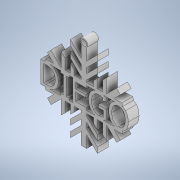
# Autodesk Inventor part: Diego
Saved by Autodesk Inventor 2021 (Build 250183000, 183)
## iProperties
Created: 2020-12-16
Part Number: Diego
Material: Genérico
Document SubType Name: Modeling
Designer: yosaf
Density: 1 g/cm^3
Appearance: Valor por defecto
Author: yosaf
Autodesk Inventor part; units mm, degrees
ref_plane "YZ Plane" through (0, 0, 0) normal (1, 0, 0) x (0, 1, 0)
ref_plane "XZ Plane" through (0, 0, 0) normal (0, 1, 0) x (-1, 0, 0)
ref_plane "XY Plane" through (0, 0, 0) normal (0, 0, 1) x (1, 0, 0)
sketch "Boceto1" plane through (0, 0, 0) normal (0, 1, 0) x (-1, 0, 0)
  point P0 (0, 0)
sketch "Boceto2" plane through (0, 0, 0) normal (0, 0, 1) x (1, 0, 0)
  line L0 (37.5, 0) -> (37.5, 10) construction
  line L1 (36.1421, 10) -> (0, 10)
  line L2 (37.5, 0) -> (37.5, -10) construction
  line L3 (36.1421, 10) -> (36.1421, 12.5) construction
  line L4 (-2.5, 37.5) -> (0, 37.5) construction
  line L5 (2.5, 37.5) -> (2.5, 12.5)
  line L6 (-2.5, 37.5) -> (-2.5, 37.4166)
  line L7 (-2.5, 37.5) -> (-2.5, 29.5) construction
  line L8 (-2.5, 29.5) -> (-9.3227, 36.3227) construction
  line L9 (-2.5, 29.5) -> (7.1487, 29.5) construction
  line L10 (-2.5, 29.5) -> (-2.5, 24.5) construction
  line L11 (2.3244, 29.5) -> (9.1827, 36.3583)
  line L12 (2.3244, 29.5) -> (12.0235, 29.5) construction
  line L13 (2.5, 24.5) -> (12.505, 34.505)
  line L14 (2.5, 12.5) -> (2.5, 14.5) construction
  line L15 (2.5, 14.5) -> (12.505, 24.505)
  line L16 (2.5, 14.5) -> (19.9142, 14.5) construction
  line L17 (12.505, 34.505) -> (12.505, 24.505) construction
  line L18 (2.5, 14.5) -> (2.5, 19.5) construction
  line L19 (2.5, 19.5) -> (9.655, 26.655)
  line L20 (9.1827, 36.3583) -> (12.505, 39.6807)
  line L21 (12.505, 39.6807) -> (12.505, 34.505)
  line L22 (9.655, 26.655) -> (12.505, 29.505)
  line L23 (12.505, 24.505) -> (12.505, 29.505)
  line L24 (12.505, 12.5) -> (12.505, 20.7373)
  line L25 (12.505, 12.5) -> (8.969, 12.5) construction
  line L26 (8.9413, 12.2486) -> (8.9413, 17.1736)
  line L27 (2.5, 37.4166) -> (2.5, 40.7545)
  line L28 (2.5, 40.7545) -> (0, 40.7545)
  line L29 (-2.5, 37.5) -> (-2.5, 37.4166)
  line L30 (12.505, 12.5) -> (17.505, 12.5) construction
  line L31 (12.505, 29.505) -> (26.5274, 43.5274) construction
  line L32 (17.505, 12.5) -> (21.041, 12.5) construction
  line L33 (21.041, 12.5) -> (21.041, 24.5)
  line L34 (21.041, 12.5) -> (27.7806, 19.2396) construction
  line L35 (21.041, 12.5) -> (21.041, 21.5913) construction
  line L36 (21.041, 12.5) -> (30.3882, 21.8472)
  line L37 (30.3882, 21.8472) -> (33.9237, 18.3116)
  arc A0 (36.1421, 10) -> (35.3553, 12.5) centre (0, 0) ccw
  line L38 (2.5, 14.5) -> (18.1273, 30.1273) construction
  line L39 (17.505, 12.5) -> (17.505, 22.0456)
  line L40 (17.505, 20.7373) -> (12.505, 20.7373) construction
  line L41 (12.505, 20.7373) -> (8.9413, 17.1736)
  line L42 (0, 40.7545) -> (0, 10) construction
  line L43 (35.3553, 12.5) -> (0, 12.5)
  line L44 (-2.5, 24.5) -> (-2.5878, 24.5878)
  line L45 (0, 10) -> (-36.142, 10)
  line L46 (0, 40.7545) -> (-2.5, 40.7545)
  line L47 (-2.5, 40.7545) -> (-2.5, 12.5)
  line L48 (-2.5, 12.5) -> (0, 12.5)
  arc A1 (10.5574, 39.7112) -> (12.505, 39.6807) centre (11.546, 40.6397) ccw construction
  line L49 (-2.505, 29.505) -> (-12.7112, 39.7112)
  line L50 (-2.505, 29.505) -> (11.9286, 29.505) construction
  line L51 (-2.5, 19.4405) -> (-12.5645, 29.505)
  line L52 (-2.5, 19.4405) -> (11.7334, 19.4405) construction
  line L53 (-12.5645, 29.505) -> (-12.5645, 24.4414)
  line L54 (-12.5645, 24.4414) -> (-2.5, 14.3769)
  line L55 (-12.5645, 12.5) -> (-2.5, 12.5)
  line L56 (17.505, 22.0456) -> (21.041, 25.5816)
  line L57 (17.505, 22.0456) -> (22.5057, 22.0456) construction
  line L58 (21.041, 25.5816) -> (21.041, 24.5)
  line L59 (-12.5645, 20.7373) -> (-12.5645, 20.7373)
  line L60 (-12.5645, 20.7373) -> (-7.5226, 20.7373) construction
  line L61 (0, 12.5) -> (-35.355, 12.5)
  arc A2 (-35.3554, 12.4999) -> (-36.1419, 10) centre (0.0007, 0.0021) ccw
  line L62 (-12.5806, 20.7428) -> (-9.0285, 17.1736)
  line L63 (-12.5645, 20.7373) -> (-17.5614, 12.5) construction
  line L64 (-17.5614, 12.5) -> (-17.5645, 22.0456)
  line L65 (-17.5645, 22.0456) -> (-21.1198, 25.6009)
  line L66 (-17.5645, 22.0456) -> (-12.5366, 22.0456) construction
  line L67 (-21.1198, 25.6009) -> (-21.1198, 12.5)
  line L68 (33.9237, 18.3116) -> (-56.2408, 18.3116) construction
  line L69 (30.1897, 22.0456) -> (-56.2408, 22.0456) construction
  line L70 (33.9237, 18.3116) -> (33.178, 17.4812)
  line L71 (33.9237, 18.3116) -> (28.1121, 12.5)
  line L72 (33.9237, 18.3116) -> (42.1426, 18.3116) construction
  line L73 (-21.1198, 12.5) -> (-30.6654, 22.0456)
  line L74 (-21.1198, 12.5) -> (-7.6202, 12.5) construction
  line L75 (-30.6654, 22.0456) -> (-33.9907, 18.3116)
  line L76 (-21.1198, 12.5) -> (-25.4451, 12.5) construction
  line L77 (-28.1908, 12.5) -> (-33.9907, 18.3116)
  line L78 (-25.4451, 12.5) -> (-25.4451, 10)
  line L79 (-2.5, 12.5) -> (-2.5, 10)
  line L80 (-12.5645, 12.5) -> (-12.5645, 10)
  line L81 (2.5, 12.5) -> (2.5, 10)
  line L82 (17.505, 12.5) -> (17.505, 10)
  line L83 (28.1121, 12.5) -> (28.1121, 10)
  line L84 (-28.1908, 12.5) -> (-28.1908, 10)
  line L85 (-36.1419, 10) -> (-35.3553, 12.5)
  line L86 (-35.3553, 12.5) -> (-28.1908, 12.5)
  line L87 (-36.1419, 10) -> (-28.1908, 10)
  line L88 (-12.5806, 20.7428) -> (-8.8604, 20.7373) construction
  line L89 (-12.5645, 24.4414) -> (-12.5645, 20.7373) construction
  line L90 (-12.5645, 20.7373) -> (-12.5645, 12.5)
  line L91 (8.9413, 17.1736) -> (-10.7205, 17.1736) construction
  line L92 (-12.5645, 12.5) -> (-9.0285, 12.5) construction
  line L93 (-9.0285, 12.4865) -> (-9.0285, 17.1736)
  line L94 (-9.0285, 12.4865) -> (-4.3415, 12.4865) construction
  line L95 (-12.5645, 12.5) -> (-17.5645, 12.5) construction
  line L96 (-17.5645, 12.5) -> (-21.1005, 12.5) construction
  line L97 (12.505, 39.6807) -> (-23.2825, 39.6807) construction
  line L98 (12.505, 39.6807) -> (48.2925, 39.6807) construction
  line L99 (-12.6807, 39.6807) -> (-12.6807, 31.9273) construction
  line L100 (-12.6807, 39.6807) -> (-4.9273, 39.6807) construction
  line L101 (2.5, 24.5) -> (-2.5, 24.5) construction
  line L102 (-2.5, 24.5) -> (-12.6807, 34.6807)
  line L103 (-12.6807, 39.6807) -> (-12.6807, 34.6807)
  line L104 (-2.5, 29.5) -> (-2.5, 24.5)
  line L105 (-12.6807, 39.6807) -> (-12.6807, 34.6807)
  line L106 (-12.6807, 34.6807) -> (-2.5, 24.5)
  line L107 (-2.5, 24.5) -> (-2.5, 29.5)
  line L108 (-5.3887, 32.3887) -> (-7.0094, 29.0094)
  line L109 (-9.8604, 36.8604) -> (-11.5, 33.5)
  line L110 (-3.3099, 30.3099) -> (-3.3099, 25.3099)
  line L111 (-3.3099, 27) -> (-2.5, 27)
  line L112 (-3.3099, 28.6951) -> (-2.5, 28.6951)
  line L113 (-2.5, 29.5) -> (-3.3099, 30.3099)
  line L114 (-3.3099, 28.6951) -> (-2.5, 28.6951)
  line L115 (-62.0182, 0.0021) -> (57.1522, 0.0021) construction
  line L116 (36.1421, -9.9958) -> (0, -9.9958)
  line L117 (36.1421, -9.9958) -> (36.1421, -12.4958) construction
  line L118 (-2.5, -37.4958) -> (0, -37.4958) construction
  line L119 (2.5, -37.4958) -> (2.5, -12.4958)
  line L120 (-2.5, -37.4958) -> (-2.5, -37.4124)
  line L121 (-2.5, -37.4958) -> (-2.5, -29.4958) construction
  line L122 (-2.5, -29.4958) -> (-9.3227, -36.3185) construction
  line L123 (-2.5, -29.4958) -> (7.1487, -29.4958) construction
  line L124 (-2.5, -29.4958) -> (-2.5, -24.4958) construction
  line L125 (2.3244, -29.4958) -> (9.1827, -36.3541)
  line L126 (2.3244, -29.4958) -> (12.0235, -29.4958) construction
  line L127 (2.5, -24.4958) -> (12.505, -34.5008)
  line L128 (2.5, -12.4958) -> (2.5, -14.4958) construction
  line L129 (2.5, -14.4958) -> (12.505, -24.5008)
  line L130 (2.5, -14.4958) -> (19.9142, -14.4958) construction
  line L131 (12.505, -34.5008) -> (12.505, -24.5008) construction
  line L132 (2.5, -14.4958) -> (2.5, -19.4958) construction
  line L133 (2.5, -19.4958) -> (9.655, -26.6507)
  line L134 (9.1827, -36.3541) -> (12.505, -39.6765)
  line L135 (12.505, -39.6765) -> (12.505, -34.5008)
  line L136 (9.655, -26.6507) -> (12.505, -29.5008)
  line L137 (12.505, -24.5008) -> (12.505, -29.5008)
  line L138 (12.505, -12.4958) -> (12.505, -20.7331)
  line L139 (12.505, -12.4958) -> (8.969, -12.4958) construction
  line L140 (8.9413, -12.2444) -> (8.9413, -17.1694)
  line L141 (2.5, -37.4124) -> (2.5, -40.7503)
  line L142 (2.5, -40.7503) -> (0, -40.7503)
  line L143 (-2.5, -37.4958) -> (-2.5, -37.4124)
  line L144 (12.505, -12.4958) -> (17.505, -12.4958) construction
  line L145 (12.505, -29.5008) -> (26.5274, -43.5232) construction
  line L146 (17.505, -12.4958) -> (21.041, -12.4958) construction
  line L147 (21.041, -12.4958) -> (21.041, -24.4958)
  line L148 (21.041, -12.4958) -> (27.7806, -19.2354) construction
  line L149 (21.041, -12.4958) -> (21.041, -21.5871) construction
  line L150 (21.041, -12.4958) -> (30.3882, -21.843)
  line L151 (30.3882, -21.843) -> (33.9237, -18.3074)
  arc A3 (35.3553, -12.4958) -> (36.1421, -9.9958) centre (0, 0.0042) ccw
  line L152 (2.5, -14.4958) -> (18.1273, -30.1231) construction
  line L153 (17.505, -12.4958) -> (17.505, -22.0414)
  line L154 (17.505, -20.7331) -> (12.505, -20.7331) construction
  line L155 (12.505, -20.7331) -> (8.9413, -17.1694)
  line L156 (0, -40.7503) -> (0, -9.9958) construction
  line L157 (35.3553, -12.4958) -> (0, -12.4958)
  line L158 (-2.5, -24.4958) -> (-2.5878, -24.5836)
  line L159 (0, -9.9958) -> (-36.142, -9.9958)
  line L160 (0, -40.7503) -> (-2.5, -40.7503)
  line L161 (-2.5, -40.7503) -> (-2.5, -12.4958)
  line L162 (-2.5, -12.4958) -> (0, -12.4958)
  arc A4 (12.505, -39.6765) -> (10.5574, -39.707) centre (11.546, -40.6355) ccw construction
  line L163 (-2.505, -29.5008) -> (-12.7112, -39.707)
  line L164 (-2.505, -29.5008) -> (11.9286, -29.5008) construction
  line L165 (-2.5, -19.4363) -> (-12.5645, -29.5008)
  line L166 (-2.5, -19.4363) -> (11.7334, -19.4363) construction
  line L167 (-12.5645, -29.5008) -> (-12.5645, -24.4372)
  line L168 (-12.5645, -24.4372) -> (-2.5, -14.3727)
  line L169 (-12.5645, -12.4958) -> (-2.5, -12.4958)
  line L170 (17.505, -22.0414) -> (21.041, -25.5774)
  line L171 (17.505, -22.0414) -> (22.5057, -22.0414) construction
  line L172 (21.041, -25.5774) -> (21.041, -24.4958)
  line L173 (-12.5645, -20.7331) -> (-12.5645, -20.7331)
  line L174 (-12.5645, -20.7331) -> (-7.5226, -20.7331) construction
  line L175 (0, -12.4958) -> (-35.355, -12.4958)
  arc A5 (-36.1419, -9.9958) -> (-35.3554, -12.4957) centre (0.0007, 0.0021) ccw
  line L176 (-12.5806, -20.7386) -> (-9.0285, -17.1694)
  line L177 (-12.5645, -20.7331) -> (-17.5614, -12.4958) construction
  line L178 (-17.5614, -12.4958) -> (-17.5645, -22.0414)
  line L179 (-17.5645, -22.0414) -> (-21.1198, -25.5967)
  line L180 (-17.5645, -22.0414) -> (-12.5366, -22.0414) construction
  line L181 (-21.1198, -25.5967) -> (-21.1198, -12.4958)
  line L182 (33.9237, -18.3074) -> (33.178, -17.477)
  line L183 (33.9237, -18.3074) -> (28.1121, -12.4958)
  line L184 (33.9237, -18.3074) -> (42.1426, -18.3074) construction
  line L185 (-21.1198, -12.4958) -> (-30.6654, -22.0414)
  line L186 (-21.1198, -12.4958) -> (-7.6202, -12.4958) construction
  line L187 (-30.6654, -22.0414) -> (-33.9907, -18.3074)
  line L188 (-21.1198, -12.4958) -> (-25.4451, -12.4958) construction
  line L189 (-28.1908, -12.4958) -> (-33.9907, -18.3074)
  line L190 (-25.4451, -12.4958) -> (-25.4451, -9.9958)
  line L191 (-2.5, -12.4958) -> (-2.5, -9.9958)
  line L192 (-12.5645, -12.4958) -> (-12.5645, -9.9958)
  line L193 (2.5, -12.4958) -> (2.5, -9.9958)
  line L194 (17.505, -12.4958) -> (17.505, -9.9958)
  line L195 (28.1121, -12.4958) -> (28.1121, -9.9958)
  line L196 (-28.1908, -12.4958) -> (-28.1908, -9.9958)
  line L197 (-36.1419, -9.9958) -> (-35.3553, -12.4958)
  line L198 (-35.3553, -12.4958) -> (-28.1908, -12.4958)
  line L199 (-36.1419, -9.9958) -> (-28.1908, -9.9958)
  line L200 (-12.5806, -20.7386) -> (-8.8604, -20.7331) construction
  line L201 (-12.5645, -24.4372) -> (-12.5645, -20.7331) construction
  line L202 (-12.5645, -20.7331) -> (-12.5645, -12.4958)
  line L203 (8.9413, -17.1694) -> (-10.7205, -17.1694) construction
  line L204 (-12.5645, -12.4958) -> (-9.0285, -12.4958) construction
  line L205 (-9.0285, -12.4823) -> (-9.0285, -17.1694)
  line L206 (-9.0285, -12.4823) -> (-4.3415, -12.4823) construction
  line L207 (-12.5645, -12.4958) -> (-17.5645, -12.4958) construction
  line L208 (-17.5645, -12.4958) -> (-21.1005, -12.4958) construction
  line L209 (12.505, -39.6765) -> (-23.2825, -39.6765) construction
  line L210 (-12.6807, -39.6765) -> (-12.6807, -31.9231) construction
  line L211 (-12.6807, -39.6765) -> (-4.9273, -39.6765) construction
  line L212 (2.5, -24.4958) -> (-2.5, -24.4958) construction
  line L213 (-2.5, -24.4958) -> (-12.6807, -34.6765)
  line L214 (-12.6807, -39.6765) -> (-12.6807, -34.6765)
  line L215 (-2.5, -29.4958) -> (-2.5, -24.4958)
  line L216 (-12.6807, -39.6765) -> (-12.6807, -34.6765)
  line L217 (-12.6807, -34.6765) -> (-2.5, -24.4958)
  line L218 (-2.5, -24.4958) -> (-2.5, -29.4958)
  line L219 (-5.3887, -32.3845) -> (-7.0094, -29.0052)
  line L220 (-9.8604, -36.8562) -> (-11.5, -33.4958)
  line L221 (-3.3099, -30.3057) -> (-3.3099, -25.3057)
  line L222 (-3.3099, -26.9958) -> (-2.5, -26.9958)
  line L223 (-3.3099, -28.6909) -> (-2.5, -28.6909)
  line L224 (-2.5, -29.4958) -> (-3.3099, -30.3057)
  line L225 (-3.3099, -28.6909) -> (-2.5, -28.6909)
  circle A6 centre (0, 43.1654) radius 3.5
  circle A7 centre (0, 43.1654) radius 2.5
  point P0 (37.5, -9.9958)
  point P1 (30.1897, -22.0414)
  point P2 (-36.1419, -9.9958)
  point P3 (-12.5645, -20.7224)
  point P4 (-9.0285, -12.4958)
  point P5 (2.5, -29.6714)
  point P6 (8.9413, -12.4958)
  point P7 (-9.0285, 12.5)
  point P8 (-12.5645, 20.7266)
  point P9 (-36.1419, 10)
  point P10 (8.9413, 12.5)
  point P11 (2.5, 29.6756)
  point P12 (-2.5, 40.7159)
  point P13 (2.5, 40.7159)
  dimension "d1" = 10
  dimension "d3" = 2.5
  dimension "d4" = 5
  dimension "d5" = 2.5
  dimension "d6" = 8
  dimension "d9" = 45
  dimension "d10" = 2
  dimension "d11" = 45
  dimension "d12" = 3.536
  dimension "d13" = 5
  dimension "d14" = 3.536
  dimension "d15" = 45
  dimension "d16" = 5
  dimension "d17" = 8
  dimension "d18" = 5.8116
  dimension "d20" = 36.1421
  dimension "d21" = 36.142
  dimension "d22" = 135
  dimension "d23" = 2.5
  dimension "d24" = 5
  dimension "d25" = 135
  dimension "d26" = 45
  dimension "d27" = 135
  dimension "d28" = 35.3553
  dimension "d29" = 35.355
  dimension "d31" = 135
  dimension "d32" = 135
  dimension "d33" = 135
  dimension "d34" = 5
  dimension "d35" = 7.071
  dimension "d36" = 3.536
  dimension "d37" = 90
  dimension "d38" = 5
  dimension "d39" = 3.536
  dimension "d40" = 180
  dimension "d41" = 90
  dimension "d42" = 8.2373
  dimension "d43" = 4.6736
  dimension "d44" = 8.2373
  dimension "d45" = 4.925
  dimension "d52" = 7
  dimension "d53" = 5
  constraints: 448 end point, 121 symmetric about line, 111 point on line, 21 horizontal, 20 perpendicular, 16 point on circle, 11 equal length, 9 vertical, 8 centre point, 7 collinear, 6 parallel, 5 midpoint, 4 coincident, 1 tangent, 23 other
  measures "d1" distance of L0.start L0.end
  measures "d3" distance of L1.start L3.end
  measures "d4" distance of L4.start L5.start
  measures "d5" horizontal distance of L5.start point (0, 0)
  measures "d6" distance of L7.end L4.start
  measures "d9" angle of L12 L11
  measures "d10" distance of L5.end L14.end
  measures "d11" angle of L16 L15
  measures "d12" distance of L24.start L25.end
  measures "d13" distance of L24.start L30.end
  measures "d14" distance of L30.end L32.end
  measures "d15" angle of L34 L35
  measures "d16" distance of L36.end L37.end
  measures "d17" vertical distance of L5.start L11.start
  measures "d20" distance of L1.start L1.end
  measures "d21" distance of L1.end L45.end
  measures "d22" angle of L50 L49
  measures "d23" distance of L46.end L28.end
  measures "d24" distance of L5.end L47.end
  measures "d25" angle of L52 L51
  measures "d26" angle of L57 L56
  measures "d27" angle of L59 L60
  measures "d28" horizontal distance of A0.end L1.end
  measures "d29" distance of L48.end L61.end
  measures "d31" angle of L66 L65
  measures "d32" angle of L71 L72
  measures "d33" angle of L74 L73
  measures "d34" distance of L73.end L75.end
  measures "d35" distance of L67.end L77.start
  measures "d36" distance of L55.start L92.end
  measures "d37" angle of L94 L93
  measures "d38" distance of L55.start L95.end
  measures "d39" distance of L95.end L96.end
  measures "d40" angle of L97 L98
  measures "d41" angle of L99 L100
  measures "d42" distance of L55.start L59.end
  measures "d43" distance of L92.end L62.end
  measures "d44" distance of L24.start L24.end
  measures "d45" distance of L26.start L26.end
  measures "d52" diameter of A6
  measures "d53" diameter of A7
sketch "Boceto3" plane through (0, 0, 0) normal (0, 0, 1) x (1, 0, 0)
  line L0 (-36.1104, 10.6812) -> (36.1378, 10.6812) construction
  line L1 (36.1378, 10.6812) -> (36.1378, -9.7992) construction
  line L2 (36.1378, -9.7992) -> (-36.1104, -9.7992) construction
  line L3 (-36.1104, -9.7992) -> (-36.1104, 10.6812) construction
  spline S0 degree 2 poles (-23.8586, -0.0173) (-23.8586, -2.8249) (-26.1346, -7.3435) (-28.045, -8.6061) knots 0 0 0 1 2 2 2
  spline S1 degree 2 poles (-28.045, -8.6061) (-29.6066, -9.5862) (-32.8129, -10.2507) (-35.3048, -10.2507) knots 0 0 0 1 2 2 2
  line L4 (-35.3048, -10.2507) -> (-40.0227, -10.2507)
  line L5 (-40.0227, -10.2507) -> (-40.0227, 10.2493)
  line L6 (-40.0227, 10.2493) -> (-35.3546, 10.2493)
  spline S2 degree 2 poles (-35.3546, 10.2493) (-32.464, 10.2493) (-29.1747, 9.3854) (-28.0118, 8.6212) knots 0 0 0 1 2 2 2
  spline S3 degree 2 poles (-28.0118, 8.6212) (-26.0349, 7.3088) (-23.8586, 2.973) (-23.8586, -0.0173) knots 0 0 0 1 2 2 2
  spline S4 degree 2 poles (-26.6994, 0.0159) (-26.6994, 2.3749) (-28.261, 5.714) (-29.806, 6.661) knots 0 0 0 1 2 2 2
  spline S5 degree 2 poles (-29.806, 6.661) (-30.9024, 7.3088) (-33.3777, 7.8903) (-35.2217, 7.8903) knots 0 0 0 1 2 2 2
  line L7 (-35.2217, 7.8903) -> (-37.2983, 7.8903)
  line L8 (-37.2983, 7.8903) -> (-37.2983, -7.8917)
  line L9 (-37.2983, -7.8917) -> (-35.2217, -7.8917)
  spline S6 degree 2 poles (-35.2217, -7.8917) (-33.4109, -7.8917) (-30.6698, -7.3103) (-29.5568, -6.5295) knots 0 0 0 1 2 2 2
  spline S7 degree 2 poles (-29.5568, -6.5295) (-28.1281, -5.5659) (-26.6994, -2.3763) (-26.6994, 0.0159) knots 0 0 0 1 2 2 2
  line L10 (-13.7582, -10.2507) -> (-21.699, -10.2507)
  line L11 (-21.699, -10.2507) -> (-21.699, -8.1575)
  line L12 (-21.699, -8.1575) -> (-19.0908, -8.1575)
  line L13 (-19.0908, -8.1575) -> (-19.0908, 8.1561)
  line L14 (-19.0908, 8.1561) -> (-21.699, 8.1561)
  line L15 (-21.699, 8.1561) -> (-21.699, 10.2493)
  line L16 (-21.699, 10.2493) -> (-13.7582, 10.2493)
  line L17 (-13.7582, 10.2493) -> (-13.7582, 8.1561)
  line L18 (-13.7582, 8.1561) -> (-16.3663, 8.1561)
  line L19 (-16.3663, 8.1561) -> (-16.3663, -8.1575)
  line L20 (-16.3663, -8.1575) -> (-13.7582, -8.1575)
  line L21 (-13.7582, -8.1575) -> (-13.7582, -10.2507)
  line L22 (-10.3858, -10.2507) -> (-10.3858, 10.2493)
  line L23 (-10.3858, 10.2493) -> (2.4392, 10.2493)
  line L24 (2.4392, 10.2493) -> (2.4392, 7.8238)
  line L25 (2.4392, 7.8238) -> (-7.6613, 7.8238)
  line L26 (-7.6613, 7.8238) -> (-7.6613, 2.2088)
  line L27 (-7.6613, 2.2088) -> (1.7581, 2.2088)
  line L28 (1.7581, 2.2088) -> (1.7581, -0.2167)
  line L29 (1.7581, -0.2167) -> (-7.6613, -0.2167)
  line L30 (-7.6613, -0.2167) -> (-7.6613, -7.8253)
  line L31 (-7.6613, -7.8253) -> (2.4392, -7.8253)
  line L32 (2.4392, -7.8253) -> (2.4392, -10.2507)
  line L33 (2.4392, -10.2507) -> (-10.3858, -10.2507)
  spline S8 degree 2 poles (14.0182, -10.6494) (11.8419, -10.6494) (8.237, -9.3204) (6.9412, -7.9748) knots 0 0 0 1 2 2 2
  spline S9 degree 2 poles (6.9412, -7.9748) (5.6454, -6.6125) (4.2666, -2.5923) (4.2666, 0.0159) knots 0 0 0 1 2 2 2
  spline S10 degree 2 poles (4.2666, 0.0159) (4.2666, 2.4912) (5.662, 6.4118) (6.9578, 7.8072) knots 0 0 0 1 2 2 2
  spline S11 degree 2 poles (6.9578, 7.8072) (8.2038, 9.1529) (11.8585, 10.6148) (14.0348, 10.6148) knots 0 0 0 1 2 2 2
  spline S12 degree 2 poles (14.0348, 10.6148) (15.0814, 10.6148) (16.9752, 10.3157) (17.8391, 10.0499) knots 0 0 0 1 2 2 2
  spline S13 degree 2 poles (17.8391, 10.0499) (18.5368, 9.8506) (20.2313, 9.1196) (20.7463, 8.8538) knots 0 0 0 1 2 2 2
  line L34 (20.7463, 8.8538) -> (20.7463, 5.5645)
  line L35 (20.7463, 5.5645) -> (20.5137, 5.5645)
  spline S14 degree 2 poles (20.5137, 5.5645) (19.9987, 6.0131) (18.9189, 6.8271) (17.9222, 7.2922) knots 0 0 0 1 2 2 2
  spline S15 degree 2 poles (17.9222, 7.2922) (17.0915, 7.7076) (14.9485, 8.2558) (13.7192, 8.2558) knots 0 0 0 1 2 2 2
  spline S16 degree 2 poles (13.7192, 8.2558) (10.7621, 8.2558) (7.1073, 3.8036) (7.1073, 0.099) knots 0 0 0 1 2 2 2
  spline S17 degree 2 poles (7.1073, 0.099) (7.1073, -1.961) (8.0709, -5.051) (8.9845, -6.1142) knots 0 0 0 1 2 2 2
  spline S18 degree 2 poles (8.9845, -6.1142) (9.865, -7.1774) (12.3569, -8.2904) (13.9185, -8.2904) knots 0 0 0 1 2 2 2
  spline S19 degree 2 poles (13.9185, -8.2904) (15.0648, -8.2904) (17.3573, -7.9582) (18.1381, -7.6259) knots 0 0 0 1 2 2 2
  line L36 (18.1381, -7.6259) -> (18.1381, -2.3265)
  line L37 (18.1381, -2.3265) -> (13.3869, -2.3265)
  line L38 (13.3869, -2.3265) -> (13.3869, 0.0657)
  line L39 (13.3869, 0.0657) -> (20.8294, 0.0657)
  line L40 (20.8294, 0.0657) -> (20.8294, -8.8885)
  spline S20 degree 2 poles (20.8294, -8.8885) (20.3144, -9.1211) (18.5534, -9.8354) (17.8059, -10.0514) knots 0 0 0 1 2 2 2
  spline S21 degree 2 poles (17.8059, -10.0514) (16.7925, -10.3504) (15.1645, -10.6494) (14.0182, -10.6494) knots 0 0 0 1 2 2 2
  spline S22 degree 2 poles (38.7544, 7.9069) (39.9173, 6.5447) (41.2131, 2.5576) (41.2131, -0.0007) knots 0 0 0 1 2 2 2
  spline S23 degree 2 poles (41.2131, -0.0007) (41.2131, -2.4926) (39.9505, -6.5295) (38.7544, -7.8917) knots 0 0 0 1 2 2 2
  spline S24 degree 2 poles (38.7544, -7.8917) (37.4918, -9.3204) (34.1527, -10.6826) (32.1426, -10.6826) knots 0 0 0 1 2 2 2
  spline S25 degree 2 poles (32.1426, -10.6826) (30.066, -10.6826) (26.7435, -9.2706) (25.5307, -7.8917) knots 0 0 0 1 2 2 2
  spline S26 degree 2 poles (25.5307, -7.8917) (24.3512, -6.5295) (23.0887, -2.5258) (23.0887, -0.0007) knots 0 0 0 1 2 2 2
  spline S27 degree 2 poles (23.0887, -0.0007) (23.0887, 2.5742) (24.3679, 6.4948) (25.5474, 7.9069) knots 0 0 0 1 2 2 2
  spline S28 degree 2 poles (25.5474, 7.9069) (26.7435, 9.2691) (30.0826, 10.6812) (32.1426, 10.6812) knots 0 0 0 1 2 2 2
  spline S29 degree 2 poles (32.1426, 10.6812) (34.2358, 10.6812) (37.5915, 9.2193) (38.7544, 7.9069) knots 0 0 0 1 2 2 2
  spline S30 degree 2 poles (38.3723, -0.0007) (38.3723, 2.026) (37.4918, 5.1658) (36.6944, 6.1958) knots 0 0 0 1 2 2 2
  spline S31 degree 2 poles (36.6944, 6.1958) (35.8804, 7.259) (33.5879, 8.3222) (32.1592, 8.3222) knots 0 0 0 1 2 2 2
  spline S32 degree 2 poles (32.1592, 8.3222) (30.6807, 8.3222) (28.4546, 7.2922) (27.6073, 6.1958) knots 0 0 0 1 2 2 2
  spline S33 degree 2 poles (27.6073, 6.1958) (26.7933, 5.1492) (25.9294, 1.9928) (25.9294, -0.0007) knots 0 0 0 1 2 2 2
  spline S34 degree 2 poles (25.9294, -0.0007) (25.9294, -4.0376) (29.3184, -8.3236) (32.1592, -8.3236) knots 0 0 0 1 2 2 2
  spline S35 degree 2 poles (32.1592, -8.3236) (34.9999, -8.3236) (38.3723, -4.0376) (38.3723, -0.0007) knots 0 0 0 1 2 2 2
  point P0 (0, 0)
  constraints: 2 other
extrude "Extrusión3" add sketch "Boceto2" along normal blind 10 contours L1 L83 L43 A0 | L1 L82 L43 L83 | L1 L81 L43 L82 | L43 L36 L37 L71 | L1 L45 L79 L48 L43 L81 | L39 L56 L58 L33 L43 | L43 L48 L47 L6 A6 L27 L5 | L43 L26 L41 L24 | L45 L80 L55 L79 | L5 L19 L22 L23 L15 | L45 L78 L61 L80 | L45 L84 L61 L78 | L90 L62 L93 L55 | L54 L53 L51 L47 | L5 L11 L20 L21 L13 | L45 L85 L61 L84 | L61 L77 L75 L73 | L61 L67 L65 L64 | L44 L102 L110 L111 L47 | L111 L110 L112 L47 | L102 L108 L49 L110 | L112 L110 L49 L113 L47 | A6 L47 L46 A7 L28 L27 | L27 L28 A7 L46 L47 A6 | L102 L109 L49 L108 | L102 L103 L49 L109 | A3 L157 L195 L116 | L195 L157 L194 L116 | L194 L157 L193 L116 | L183 L151 L150 L157 | L193 L157 L162 L191 L159 L116 | L157 L147 L172 L170 L153 | L119 L141 L142 L160 L161 L120 L162 L157 | L138 L155 L140 L157 | L191 L169 L192 L159 | L129 L137 L136 L133 L119 | L192 L175 L190 L159 | L190 L175 L196 L159 | L169 L205 L176 L202 | L161 L165 L167 L168 | L127 L135 L134 L125 L119 | L196 L175 L197 L159 | L175 L185 L187 L189 | L178 L179 L181 L175 | L161 L222 L221 L213 L158 | L161 L223 L221 L222 | L221 L163 L219 L213 | L161 L224 L163 L221 L223 | L219 L163 L220 L213 | L220 L163 L214 L213
extrude "Extrusión4" add sketch "Boceto3" along normal blind 10
